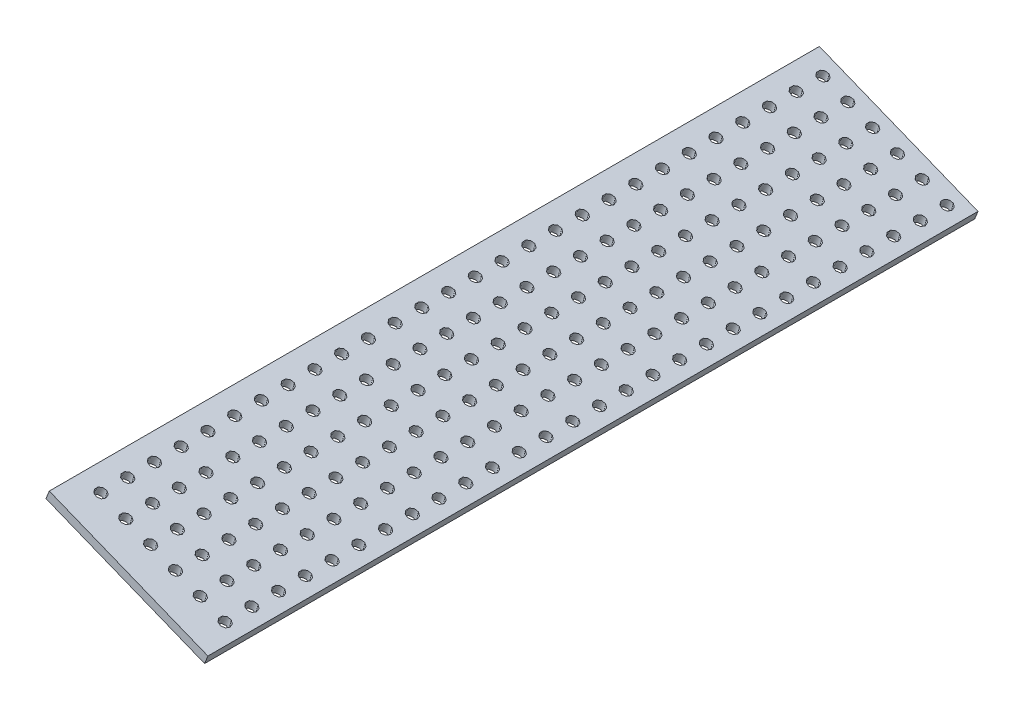
# Autodesk Inventor part: platte3
Saved by Autodesk Inventor 2023 (Build 270158000, 158)
## iProperties
Created: 2022-09-26
Part Number: platte3
Material: Generic
Document SubType Name: Modeling
Designer: bananenbrot
Density: 1 g/cm^3
Appearance: Default
Author: bananenbrot
Autodesk Inventor part; units mm, degrees
ref_plane "YZ Plane" through (0, 0, 0) normal (1, 0, 0) x (0, 1, 0)
ref_plane "XZ Plane" through (0, 0, 0) normal (0, 1, 0) x (-1, 0, 0)
ref_plane "XY Plane" through (0, 0, 0) normal (0, 0, 1) x (1, 0, 0)
sketch "Sketch1" plane through (0, 0, 0) normal (0, 0, 1) x (1, 0, 0)
  line L0 (30.2718, -10.3509) -> (29.0445, -13.4142) projected
  line L1 (-30.2718, 10.3509) -> (-29.0445, 13.4142) projected
  line L2 (-29.0445, 13.4142) -> (30.2718, -10.3509)
  line L3 (29.0445, -13.4142) -> (-30.2718, 10.3509)
  point P0 (0, 0)
  constraints: 4 end point, 1 perpendicular
extrude "Extrusion1" add sketch "Sketch1" along normal blind 288
sketch "Sketch2" plane through (-29.0445, 13.4142, 288) normal (0.3719097, 0.9282689, 0) x (0.9282689, -0.3719097, 0)
  line L0 (63.9, 288) -> (0, 288) projected
  line L1 (0, 288) -> (0, 0) projected
  line L2 (63.9, 0) -> (0, 0) projected
  line L3 (63.9, 288) -> (63.9, 0) projected
  circle A0 centre (57.9, 282) radius 2
  point P0 (31.95, 288)
  dimension "d2" = 4
  dimension "d3" = 6
  dimension "d4" = 6
  constraints: 1 centre point
  measures "d2" diameter of A0
  measures "d3" distance from line of L3 A0.centre
  measures "d4" distance from line of L0 A0.centre
extrude "Extrusion2" cut sketch "Sketch2" against normal blind 288 contours A0
pattern_linear "Rectangular Pattern1" count 28 spacing 10 along (0, 0, 1) count 6 spacing 10 along (-0.9282689, 0.3719097, 0) of "Extrusion2"
body "Solid1"
